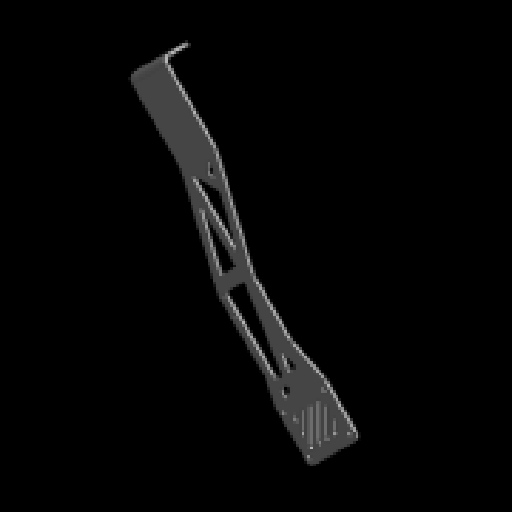
# Autodesk Inventor part: ArmScapulaLong
Saved by Autodesk Inventor 2025.2 (Build 292293000, 293)
## iProperties
Created: 2025-02-16
Part Number: ArmScapulaLong
Material: Generic
Document SubType Name: Sheet Metal
Designer: valer
Density: 1 g/cm^3
Appearance: Default
Sheet Metal Rule: Default
Author: valer
Autodesk Inventor part; units mm, degrees
ref_plane "YZ Plane" through (0, 0, 0) normal (1, 0, 0) x (0, 1, 0)
ref_plane "XZ Plane" through (0, 0, 0) normal (0, 1, 0) x (-1, 0, 0)
ref_plane "XY Plane" through (0, 0, 0) normal (0, 0, 1) x (1, 0, 0)
sketch "Base" plane through (0, 0, 0) normal (0, 0, 1) x (1, 0, 0)
  line L0 (-56.5685, 84.8528) -> (-77.6161, 135.6662)
  line L1 (-117.6161, 135.6662) -> (-84.8528, 56.5685)
  line L2 (-84.8528, 56.5685) -> (-14.1421, -14.1421)
  line L3 (-56.5685, 84.8528) -> (-84.8528, 56.5685) construction
  line L4 (-34.9925, 44.5247) -> (-17.1673, 36.9663)
  line L5 (-17.1673, 36.9663) -> (-25.5183, 28.6152)
  line L6 (-25.5183, 28.6152) -> (-34.9925, 44.5247)
  line L7 (-62.4745, 78.9469) -> (-80.6102, 60.8112)
  line L8 (-80.6102, 60.8112) -> (-36.9663, 17.1673)
  line L9 (-67.0923, 110.2595) -> (-101.2345, 96.1174) construction
  line L10 (-62.4745, 78.9469) -> (-29.8952, 24.2383)
  line L11 (-29.8952, 24.2383) -> (-36.9663, 17.1673)
  line L12 (-79.9683, 125.6662) -> (-65.3029, 90.2606)
  line L13 (-65.3029, 90.2606) -> (-84.4027, 71.1607)
  line L14 (-84.4027, 71.1607) -> (-106.9796, 125.6662)
  line L15 (-106.9796, 125.6662) -> (-79.9683, 125.6662)
  line L16 (-25.5183, 28.6152) -> (-29.8952, 24.2383) construction
  line L17 (-56.5685, 84.8528) -> (14.1421, 14.1421)
  line L18 (-69.5455, 86.018) -> (-105.414, 121.8865)
  line L19 (-65.3029, 90.2606) -> (-100.7085, 125.6662)
  line L20 (-77.6161, 135.6662) -> (-117.6161, 135.6662)
  line L21 (-14.1421, -14.1421) -> (14.1421, 14.1421)
  line L22 (-62.4745, 78.9469) -> (-69.5455, 86.018)
  point P0 (0, 0)
  point P1 (-72.6356, 107.9634)
  point P2 (-104.5743, 121.0468)
  point P3 (0, 0)
  dimension "d8" = 6
  dimension "d9" = 6
  dimension "d22" = 10
  dimension "d23" = 6
  dimension "d29" = 55
  dimension "d30" = 10
  dimension "d79" = 6
  dimension "d124" = 67.978
  dimension "d125" = 6
  dimension "d198" = 6
  dimension "d199" = 100
  dimension "d200" = 14.226
  dimension "d201" = 36.9552
  dimension "d202" = 157.5
  dimension "d203" = 40
  measures "d8" distance between parallel lines of L1 L14
  measures "d9" distance between parallel lines of L0 L12
  measures "d22" distance between parallel lines of L7 L13
  measures "d23" distance from line of L17 L4.end
  measures "d29" distance of L0.start L0.end
  measures "d30" distance of L10.end L8.end
  measures "d79" distance between parallel lines of L18 L19
  measures "d124" angle of L5 L4
  measures "d125" distance between parallel lines of L10 L6
  measures "d198" distance between parallel lines of L2 L8
  measures "d199" distance of L0.start L17.end
  measures "d200" angle of L8 L10
  measures "d201" distance of L9.start L9.end
  measures "d202" angle of L0 L17
  measures "d203" distance of L2.end L17.end
extrude "Plate1" add sketch "Base" along normal blind 3.048 contours L17 L21 L2 L1 L20 L0 | L13 L18 L14 L15 L19
delete faces "Delete1" heal yes whole lump no faces at (-93.7951, 125.6662, 1.016)
fillet "InsideFilletsFeature" radius 2 10 edges at (-17.1673, 36.9663, 1.524) (-25.5183, 28.6152, 1.524) (-34.9925, 44.5247, 1.524) (-36.9663, 17.1673, 1.524) (-29.8952, 24.2383, 1.524) (-62.4745, 78.9469, 1.524) (-80.6102, 60.8112, 1.524) (-84.4027, 71.1607, 1.524) (-65.3029, 90.2606, 1.524) (-105.414, 121.8865, 1.524)
sketch "Mount" plane through (-77.6161, 135.6662, 0) normal (0, 0, -1) x (-1, 0, 0)
  arc A0 (-84.819, -103.9794) -> (-83.1169, -102.2772) centre (-83.2002, -103.896) ccw construction
  arc A1 (-106.7394, -125.8997) -> (-105.0372, -124.1975) centre (-105.1205, -125.8163) ccw construction
  arc A2 (-46.9331, -138.4609) -> (-48.6353, -140.1631) centre (-48.552, -138.5443) ccw construction
  arc A3 (-68.8534, -160.3813) -> (-70.5556, -162.0834) centre (-70.4723, -160.4646) ccw construction
  line L0 (-63.474, -149.8083) -> (-91.7583, -121.5241)
  line L1 (-63.474, -149.8083) -> (7.2367, -79.0976)
  line L2 (-33.2934, -119.6277) -> (-41.688, -137.6301)
  line L3 (-41.688, -137.6301) -> (-71.3865, -167.3285)
  line L4 (-71.3865, -167.3285) -> (-112.1916, -126.5234)
  line L5 (-112.1916, -126.5234) -> (-82.4931, -96.825)
  line L6 (-82.4931, -96.825) -> (-53.574, -83.3398)
  line L7 (-91.7583, -121.5241) -> (-21.0476, -50.8134)
  line L8 (-44.1022, -138.6301) -> (-70.3865, -164.9143) construction
  line L9 (-83.4931, -99.2392) -> (-109.7774, -125.5234) construction
  line L10 (-109.7774, -128.9377) -> (-73.5936, -165.1214) construction
  circle A4 centre (-48.552, -138.5443) radius 2
  circle A5 centre (-70.4723, -160.4646) radius 2
  circle A6 centre (-83.2002, -103.896) radius 2
  circle A7 centre (-105.1205, -125.8163) radius 2
  point P0 (-77.6161, -135.6662)
sheet face with bend "MountFeature" sketch "Mount" thickness 3.048 toward (0, 0, 1) bend radius 3.048 relief straight relief width 3.048 relief depth 1.524
bend "Bend4"
fillet "OutsideFilletsFeature" radius 4 8 edges at (-6.2297, -31.6623, 1.524) (34.5754, 9.1427, 1.524) (4.877, 38.8412, 1.524) (-35.9281, -1.9639, 1.524) (-44.3228, 16.0385, 1.524) (-24.0421, 52.3264, 1.524) (-84.8528, 56.5685, 1.524) (-56.5685, 84.8528, 1.524)
sketch "VentHoles" plane through (-77.6161, 135.6662, 0) normal (0, 0, -1) x (-1, 0, 0)
  line L0 (-58.536, -135.9217) -> (-58.536, -138.9217) construction
  line L1 (-60.536, -135.9217) -> (-60.536, -138.9217)
  line L2 (-56.536, -138.9217) -> (-56.536, -135.9217)
  arc A0 (-56.536, -135.9217) -> (-60.536, -135.9217) centre (-58.536, -135.9217) ccw
  arc A1 (-60.536, -138.9217) -> (-56.536, -138.9217) centre (-58.536, -138.9217) ccw
  circle A2 centre (-48.552, -138.5443) radius 2 construction
  circle A3 centre (-105.1205, -125.8163) radius 2 construction
  line L3 (-65.3148, -145.7005) -> (-65.3148, -129.1429) construction
  line L4 (-63.3148, -145.7005) -> (-63.3148, -129.1429)
  line L5 (-67.3148, -129.1429) -> (-67.3148, -145.7005)
  arc A4 (-67.3148, -145.7005) -> (-63.3148, -145.7005) centre (-65.3148, -145.7005) ccw
  arc A5 (-63.3148, -129.1429) -> (-67.3148, -129.1429) centre (-65.3148, -129.1429) ccw
  line L6 (-72.0936, -122.3641) -> (-72.0936, -152.4793) construction
  line L7 (-74.0936, -122.3641) -> (-74.0936, -152.4793)
  line L8 (-70.0936, -152.4793) -> (-70.0936, -122.3641)
  arc A6 (-70.0936, -122.3641) -> (-74.0936, -122.3641) centre (-72.0936, -122.3641) ccw
  arc A7 (-74.0936, -152.4793) -> (-70.0936, -152.4793) centre (-72.0936, -152.4793) ccw
  circle A8 centre (-70.4723, -160.4646) radius 2 construction
  line L9 (-78.8724, -115.5852) -> (-78.8724, -145.7005) construction
  line L10 (-76.8724, -115.5852) -> (-76.8724, -145.7005)
  line L11 (-80.8724, -145.7005) -> (-80.8724, -115.5852)
  arc A9 (-76.8724, -115.5852) -> (-80.8724, -115.5852) centre (-78.8724, -115.5852) ccw
  arc A10 (-80.8724, -145.7005) -> (-76.8724, -145.7005) centre (-78.8724, -145.7005) ccw
  line L12 (-85.6512, -115.5394) -> (-85.6512, -138.9217) construction
  line L13 (-87.6512, -115.5394) -> (-87.6512, -138.9217)
  line L14 (-83.6512, -138.9217) -> (-83.6512, -115.5394)
  arc A11 (-83.6512, -115.5394) -> (-87.6512, -115.5394) centre (-85.6512, -115.5394) ccw
  arc A12 (-87.6512, -138.9217) -> (-83.6512, -138.9217) centre (-85.6512, -138.9217) ccw
  circle A13 centre (-83.2002, -103.896) radius 2 construction
  line L15 (-92.43, -132.1429) -> (-92.43, -122.3183) construction
  line L16 (-94.43, -132.1429) -> (-94.43, -122.3183)
  line L17 (-90.43, -122.3183) -> (-90.43, -132.1429)
  arc A14 (-94.43, -132.1429) -> (-90.43, -132.1429) centre (-92.43, -132.1429) ccw
  arc A15 (-90.43, -122.3183) -> (-94.43, -122.3183) centre (-92.43, -122.3183) ccw
  line L18 (-54.2075, -137.4217) -> (-72.0936, -155.3077) construction
  line L19 (-72.0936, -155.3077) -> (-100.1708, -127.2306) construction
  line L20 (-100.1708, -127.2306) -> (-82.2847, -109.3445) construction
  line L21 (-82.2847, -109.3445) -> (-54.2075, -137.4217) construction
  line L22 (-42.0641, -117.0847) -> (-46.6205, -112.5283) construction
  line L23 (-68.5581, -164.5001) -> (-42.1867, -138.1288) construction
  line L24 (-109.3631, -129.3519) -> (-74.2149, -164.5001) construction
  line L25 (-82.9918, -97.3237) -> (-109.3631, -123.695) construction
  point P0 (-77.6161, -135.6662)
  point P1 (-58.536, -137.4217)
  point P2 (-65.3148, -137.4217)
  point P3 (-72.0936, -137.4217)
  point P4 (-78.8724, -130.6429)
  point P5 (-85.6512, -127.2306)
  point P6 (-92.43, -127.2306)
  point P7 (-97.6499, -127.9377)
  dimension "d142" = 4
  dimension "d158" = 6.7788
  dimension "d159" = 6.7788
  dimension "d160" = 6.7788
  dimension "d161" = 6.7788
  dimension "d162" = 6.7788
  dimension "d164" = 9
  dimension "d165" = 8
  dimension "d166" = 9
  dimension "d167" = 8
  dimension "d168" = 45
  dimension "d170" = 3
  constraints: 56 end point, 37 tangent, 24 point on circle, 12 centre point, 12 parallel, 6 midpoint, 5 equal radius, 2 perpendicular
  measures "d142" diameter of A1
  measures "d158" distance between parallel lines of L3 L0
  measures "d159" distance between parallel lines of L6 L3
  measures "d160" distance between parallel lines of L9 L6
  measures "d161" distance between parallel lines of L12 L9
  measures "d162" distance between parallel lines of L15 L12
  measures "d164" distance between parallel lines of L23 L18
  measures "d165" distance between parallel lines of L24 L19
  measures "d166" distance between parallel lines of L25 L20
  measures "d167" distance from line of L23.end L21
  measures "d168" angle of L21 L0
  measures "d170" distance of L0.start L0.end
extrude "VentHolesFeature" cut sketch "VentHoles" against normal blind 3.048
sketch "Connector" plane through (-77.6161, 135.6662, 0) normal (0, 0, -1) x (-1, 0, 0)
  line L0 (40, 0) -> (7.5412, -78.3626)
  line L1 (-20.7431, -50.0783) -> (0, 0)
  line L2 (40, 0) -> (0, 0)
  line L3 (0, 0) -> (11.7157, 28.2843)
  line L4 (11.7157, 28.2843) -> (57.6777, 74.2462)
  line L5 (57.6777, 74.2462) -> (85.9619, 45.9619)
  line L6 (85.9619, 45.9619) -> (40, 0)
  line L7 (40, 0) -> (11.7157, 28.2843) construction
  line L8 (-68.5581, -164.5001) -> (-42.1867, -138.1288)
  point P0 (-77.6161, -135.6662)
  point P1 (25.8579, 14.1421)
  point P2 (20, 0)
  dimension "JacobiRadiusSize" = 3.048
  dimension "d177" = 65
  measures "d177" distance of L5.end L0.start
sheet face with bend "ConnectorFeature" sketch "Connector" thickness 3.048 toward (0, 0, 1) bend radius 3.048 relief straight relief width 3.048 relief depth 1.524
bend "Bend5"
sketch "Sketch18" plane through (-133.1385, 207.7571, 3.048) normal (-0.7071068, 0.7071068, 0) x (-0.7071068, -0.7071068, 0)
  line L0 (40, 0) -> (0, 0)
  line L1 (0, 0) -> (0, -25)
  line L2 (0, -25) -> (40, -25)
  line L3 (40, -25) -> (40, 0)
  constraints: 6 end point, 1 horizontal, 1 perpendicular, 1 vertical
edge flange "BodyMountFeature" height 25 angle 90 thickness 3.048 bend radius 3.048 thickness toward (-0.7071068, 0.7071068, 0) relief straight relief width 3.048 relief depth 1.524 edges at (-149.4359, 195.7703, 0) wall of the first edge with corners at (-161.4228, 179.4729, 3.048) (-133.1385, 207.7571, 3.048) (-133.1385, 207.7571, -21.952) (-161.4228, 179.4729, -21.952)
bend "Bend6"
corner "Corner4"
fillet "BodyMountFilletsFeature" radius 4 2 edges at (-162.5004, 180.5505, -21.952) (-134.2162, 208.8348, -21.952)
sketch "Sketch19" plane through (-6.2297, -26.0055, 0) normal (0, 0, -1) x (-1, 0, 0)
  line L0 (89.3347, 167.6717) -> (80.3661, 167.6717)
  line L1 (80.3661, 167.6717) -> (87.6944, 185.3638)
  line L2 (87.6944, 185.3638) -> (89.3347, 167.6717)
  line L3 (83.1022, 189.956) -> (50.6434, 111.5934) projected
  line L4 (111.3865, 161.6717) -> (83.1022, 189.956)
  line L5 (62.921, 125.5554) -> (77.8808, 161.6717) construction
  line L6 (77.8808, 161.6717) -> (104.4788, 161.6717) projected
  point P0 (-6.2297, 26.0055)
  dimension "d216" = 6
  constraints: 8 end point, 1 collinear, 1 parallel, 1 point on line
  measures "d216" distance between parallel lines of L6 L0
extrude "BodyMountCutFeature" cut sketch "Sketch19" against normal blind 3.048
fillet "BodyMountInsideFilletsFeature" radius 2 5 edges at (-95.5643, 141.6662, 1.524) (-86.5958, 141.6662, 1.524) (-93.9241, 159.3583, 1.524) (-84.1105, 135.6662, 1.524) (-110.7085, 135.6662, 1.524)
sketch "Sketch20" plane through (-163.5781, 181.6281, -17.952) normal (-0.7071068, 0.7071068, 0) x (-0.7071068, -0.7071068, 0)
  line L0 (-8, 5) -> (-32, 5) construction
  line L1 (-4, -4) -> (-36, -4) construction
  line L2 (0, 14.904) -> (0, 0) construction
  line L3 (-40, 0) -> (-40, 14.904) construction
  circle A0 centre (-8, 5) radius 3
  circle A1 centre (-32, 5) radius 3
  point P0 (12.7633, 17.952)
  dimension "d192" = 8
  dimension "d193" = 8
  dimension "d194" = 9
  dimension "d195" = 6
  constraints: 2 centre point, 2 coincident, 2 end point, 1 equal radius, 1 parallel
  measures "d192" distance from line of L2 L0.start
  measures "d193" distance from line of L3 L0.end
  measures "d194" distance between parallel lines of L1 L0
  measures "d195" diameter of A0
extrude "BodyMountHolesFeature" cut sketch "Sketch20" against normal blind 3.048
sketch "Sketch21" plane through (-6.2297, -26.0055, 0) normal (0, 0, -1) x (-1, 0, 0)
  arc A0 (13.6686, 64.1298) -> (13.0351, 60.8742) centre (14.4493, 62.2885) ccw projected
  line L0 (17.4712, 56.4382) -> (13.0351, 60.8742) projected
  line L1 (19.1091, 43.4866) -> (23.6655, 38.9301) construction
  circle A1 centre (19.1091, 43.4866) radius 2
  circle A2 centre (23.6655, 38.9301) radius 2
  line L2 (20.5233, 44.9008) -> (25.0798, 40.3443)
  line L3 (19.1091, 43.4866) -> (22.1986, 35.7842) construction
  line L4 (22.1986, 35.7842) -> (23.6655, 38.9301) construction
  circle A3 centre (22.1986, 35.7842) radius 2
  line L5 (25.4782, 38.0849) -> (24.0112, 34.939)
  line L6 (20.3423, 35.0396) -> (17.2529, 42.742)
  line L7 (13.6686, 64.1298) -> (23.1373, 68.1448) projected
  arc A4 (29.3224, 44.587) -> (32.1508, 44.587) centre (30.7366, 46.0012) ccw projected
  line L8 (23.6655, 38.9301) -> (30.7366, 46.0012) construction
  arc A5 (17.4712, 56.4382) -> (20.6038, 56.8291) centre (18.8854, 57.8524) ccw projected
  line L9 (29.3224, 44.587) -> (24.766, 49.1434) projected
  arc A6 (24.4618, 51.5809) -> (24.766, 49.1434) centre (26.1802, 50.5576) ccw projected
  line L10 (19.1091, 43.4866) -> (26.1802, 50.5576) construction
  line L11 (29.9966, 24.6809) -> (37.7951, 41.4048) projected
  line L12 (-37.9767, 32.3198) -> (-2.8284, -2.8284) projected
  line L13 (17.1733, 78.0338) -> (-10.4674, 65.1448) projected
  point P0 (-6.2297, 26.0055)
  dimension "d210" = 6
  dimension "d211" = 45
  constraints: 16 end point, 6 point on circle, 6 tangent, 3 centre point, 3 coincident, 3 equal radius, 2 parallel, 2 perpendicular
  measures "d210" distance between parallel lines of L9 L2
  measures "d211" distance from line of L12 L3.end
extrude "ExtraCutFeature" cut sketch "Sketch21" against normal blind 3.048
sketch "LimitSwitchMountHoles" plane through (-6.2297, -26.0055, 0) normal (0, 0, -1) x (-1, 0, 0)
  circle A0 centre (75.9262, 83.9972) radius 1 projected
  circle A1 centre (66.0267, 74.0977) radius 1 projected
  point P0 (-6.2297, 26.0055)
extrude "LimitSwitchMountHolesFeature" cut sketch "LimitSwitchMountHoles" against normal blind 3.048
equation "\"d22\" = 2 * d3"
equation "\"d3\" = 5"
body "Solid2"
